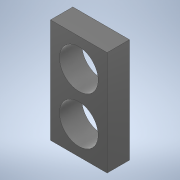
# Autodesk Inventor part: LED-Spacer1
Saved by Autodesk Inventor 2022 (Build 260153000, 153)
## iProperties
Created: 2024-06-27
Part Number: LED-Spacer1
Material: 一般
Document SubType Name: Modeling
Designer: yamashita1
Density: 1 g/cm^3
Appearance: 既定
Author: yamashita1
Autodesk Inventor part; units mm, degrees
ref_plane "YZ Plane" through (0, 0, 0) normal (1, 0, 0) x (0, 1, 0)
ref_plane "XZ Plane" through (0, 0, 0) normal (0, 1, 0) x (-1, 0, 0)
ref_plane "XY Plane" through (0, 0, 0) normal (0, 0, 1) x (1, 0, 0)
sketch "スケッチ1" plane through (0, 0, 0) normal (0, 0, 1) x (1, 0, 0)
  circle A0 centre (0, 3.8) radius 2.6
  circle A1 centre (0, 10.2) radius 2.6
  line L0 (-3.8, 0) -> (3.8, 0)
  line L1 (3.8, 0) -> (3.8, 14)
  line L2 (3.8, 14) -> (-3.8, 14)
  line L3 (-3.8, 14) -> (-3.8, 0)
  line L4 (-11.5586, 7) -> (11.5586, 7) construction
  point P0 (0, 0)
  point P1 (0, 0)
  point P2 (0, 7)
  dimension "LED_DIA" = 5.2
  dimension "d1" = 7.6
  dimension "LED_PITCH" = 6.4
  dimension "d3" = 14
  constraints: 10 end point, 2 centre point, 2 horizontal, 2 midpoint, 2 parallel, 2 vertical alignment, 1 coincident, 1 equal radius, 1 perpendicular, 1 symmetric about line, 1 other
  measures "LED_DIA" diameter of A0
  measures "d1" distance of L0.start L0.end
  measures "LED_PITCH" distance of A1.centre A0.centre
  measures "d3" distance of L0.end L1.end
extrude "スペーサ" add sketch "スケッチ1" along normal blind 3
